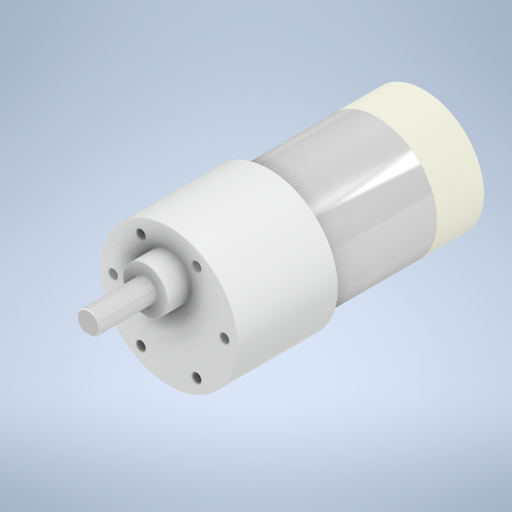
# Autodesk Inventor part: Vince-Motor
Saved by Autodesk Inventor 2024 (Build 280153000, 153)
## iProperties
Created: 2023-12-18
Part Number: Vince-Motor
Material: Generic
Document SubType Name: Modeling
Designer: greg
Density: 1 g/cm^3
Appearance: Aluminum - Flat
Author: greg
Autodesk Inventor part; units mm, degrees
ref_plane "YZ Plane" through (0, 0, 0) normal (1, 0, 0) x (0, 1, 0)
ref_plane "XZ Plane" through (0, 0, 0) normal (0, 1, 0) x (-1, 0, 0)
ref_plane "XY Plane" through (0, 0, 0) normal (0, 0, 1) x (1, 0, 0)
sketch "Sketch2" plane through (0, 0, 0) normal (1, 0, 0) x (0, 1, 0)
  line L0 (0, 0) -> (0, -90.5559) construction
  line L1 (0, 0) -> (18.5, 0)
  line L2 (18.5, 0) -> (18.5, -27)
  line L3 (18.5, -27) -> (0, -27)
  line L4 (0, -27) -> (0, 0)
  line L5 (0, -27) -> (16.15, -27)
  line L6 (16.15, -28) -> (16.15, -56)
  line L7 (16.15, -56) -> (0, -56)
  line L8 (0, -56) -> (0, -27)
  line L9 (0, -56) -> (16.16, -56)
  line L10 (16.16, -56) -> (16.16, -68.7)
  line L11 (16.16, -68.7) -> (0, -68.7)
  line L12 (0, -68.7) -> (0, -56)
  arc A0 (16.15, -28) -> (15.15, -27) centre (15.15, -28) ccw
  line L13 (16.15, -28) -> (15.15, -28) construction
  line L14 (15.15, -27) -> (15.15, -28) construction
  dimension "d1" = 27
  dimension "d3" = 41.7
  dimension "d4" = 37
  dimension "d5" = 0.01
  dimension "d6" = 2.35
  dimension "d7" = 29
  dimension "d8" = 1
  dimension "d9" = 90
  constraints: 30 end point, 6 parallel, 3 horizontal, 3 perpendicular, 2 point on circle, 1 centre point, 1 point on line, 1 tangent, 1 vertical
  measures "d1" distance of L1.end L2.end
  measures "d3" distance between parallel lines of L3 L11
  measures "d4" diameter of L2 L0
  measures "d5" distance between parallel lines of L6 L10
  measures "d6" distance between parallel lines of L2 L6
  measures "d7" distance between parallel lines of L7 L3
  measures "d8" radius of A0
  measures "d9" angle of L13 L14
revolve "Revolution1" add sketch "Sketch2" angle 360 about axis through (0, 0, 0) along (0, 0, -1)
sketch "Sketch4" plane through (0, 0, 0) normal (1, 0, 0) x (0, 1, 0)
  line L0 (7, 0) -> (7, 36.4313)
  line L1 (7, 0) -> (0, 0)
  line L2 (-18.5, 0) -> (18.5, 0) projected
  line L3 (7, 0) -> (13, 0)
  line L4 (13, 0) -> (13, 6.3)
  line L5 (13, 6.3) -> (7, 6.3)
  line L6 (7, 6.3) -> (7, 0)
  line L7 (7, 6.3) -> (10, 6.3)
  line L8 (10, 6.3) -> (10, 21.8)
  line L9 (10, 21.8) -> (7, 21.8)
  line L10 (7, 21.8) -> (7, 6.3)
  dimension "d12" = 7
  dimension "d13" = 6.3
  dimension "d14" = 12
  dimension "d15" = 15.5
  dimension "d16" = 6
  constraints: 20 end point, 4 parallel, 2 horizontal, 2 perpendicular, 1 collinear, 1 horizontal alignment, 1 vertical
  measures "d12" distance of L0.start L1.end
  measures "d13" distance of L3.end L4.end
  measures "d14" diameter of L4 L0
  measures "d15" distance of L7.end L8.end
  measures "d16" diameter of L8 L0
revolve "Revolution2" add sketch "Sketch4" angle 360 about axis through (0, 7, 0) along (0, 0, 1)
chamfer "Chamfer1" distance 0.25 angle 45 1 edges at (0, 4, 21.8)
sketch "Sketch5" plane through (0, 7, 21.8) normal (0, 0, 1) x (1, 0, 0)
  circle A0 centre (0, 0) radius 3 projected
  line L0 (-1.6583, -2.5) -> (1.6583, -2.5)
  point P0 (0, -7)
  point P1 (0, 3)
  dimension "d18" = 5.5
  constraints: 3 point on circle, 2 end point, 1 horizontal, 1 vertical alignment
  measures "d18" distance from line of L0 point (0, 3)
extrude "Extrusion1" cut sketch "Sketch5" against normal blind 12 contours L0 A0 picked at (-0.3442, -2.6056)
sketch "Sketch6" plane through (0, 0, 0) normal (0, 0, 1) x (1, 0, 0)
  point P0 (0, 0)
  point P1 (-15, 0)
  dimension "d24" = 15
  constraints: 1 horizontal alignment
  measures "d24" distance of point (0, 0) point (-15, 0)
hole "Hole1" at (-15, 0, 0) direction (0, 0, -1) diameter 2.459 depth 3.5 thread size "M3x0.5" class "6H" standard "ISO Metric profile"
pattern_circular "Circular Pattern1" count 6 over 360 about axis through (0, 0, -13.5) along (0, 0, -1) of "Hole1"
body "Solid1"
